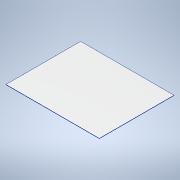
# Autodesk Inventor part: aluminiumBase
Saved by Autodesk Inventor 2020 (Build 240168000, 168)
## iProperties
Created: 2022-05-17
Part Number: aluminiumBase
Material: Aluminium 6061
Document SubType Name: Modeling
Designer: mikoma
Density: 2.7 g/cm^3
Appearance: Aluminium — płaski
Mass: 6480 g
Surface Area: 16108 cm^2
Volume: 2400 cm^3
Author: mikoma
Autodesk Inventor part; units mm, degrees
ref_plane "YZ Plane" through (0, 0, 0) normal (1, 0, 0) x (0, 1, 0)
ref_plane "XZ Plane" through (0, 0, 0) normal (0, 1, 0) x (-1, 0, 0)
ref_plane "XY Plane" through (0, 0, 0) normal (0, 0, 1) x (1, 0, 0)
sketch "Szkic1" plane through (0, 0, 0) normal (0, 1, 0) x (-1, 0, 0)
  line L0 (-500, 400) -> (500, 400)
  line L1 (500, 400) -> (500, -400)
  line L2 (500, -400) -> (-500, -400)
  line L3 (-500, -400) -> (-500, 400)
  line L4 (-500, 400) -> (500, -400) construction
  line L5 (500, 400) -> (-500, -400) construction
  point P0 (0, 0)
  dimension "d0" = 800
  dimension "d1" = 1000
  constraints: 12 end point, 2 midpoint, 2 parallel, 1 horizontal, 1 perpendicular
  measures "d0" distance between parallel lines of L2 L0
  measures "d1" distance between parallel lines of L3 L1
extrude "Wyciągnięcie proste1" add sketch "Szkic1" along normal blind 3
